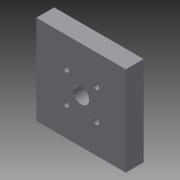
# Autodesk Inventor part: lmk8uugen
Saved by Autodesk Inventor 2014 (Build 180170000, 170)
## iProperties
Created: 2014-07-13
Part Number: lmk8uugen
Material: Generic
Document SubType Name: Modeling
Designer: cruiser
Density: 1 g/cm^3
Appearance: Default
Author: cruiser
Autodesk Inventor part; units mm, degrees
ref_plane "YZ Plane" through (0, 0, 0) normal (1, 0, 0) x (0, 1, 0)
ref_plane "XZ Plane" through (0, 0, 0) normal (0, 1, 0) x (-1, 0, 0)
ref_plane "XY Plane" through (0, 0, 0) normal (0, 0, 1) x (1, 0, 0)
sketch "Sketch1" plane through (0, 0, 0) normal (0, 1, 0) x (-1, 0, 0)
  line L0 (25, -25) -> (-25, -25)
  line L1 (-25, -25) -> (-25, 25)
  line L2 (-25, 25) -> (25, 25)
  line L3 (25, 25) -> (25, -25)
  line L4 (25, -25) -> (-25, 25) construction
  line L5 (-25, -25) -> (25, 25) construction
  point P0 (0, 0)
  dimension "d0" = 50
  dimension "d1" = 50
  constraints: 12 end point, 2 midpoint, 2 parallel, 1 horizontal, 1 perpendicular
  measures "d0" distance of L1.end L2.end
  measures "d1" distance of L0.end L1.end
extrude "Extrusion1" add sketch "Sketch1" along normal blind 10
sketch "Sketch2" plane through (0, 10, 0) normal (0, 1, 0) x (1, 0, 0)
  circle A0 centre (0, 0) radius 4.5
  circle A1 centre (8.4853, 8.4853) radius 1.65
  line L0 (0, 0) -> (8.4853, 8.4853)
  line L1 (0, 0) -> (12, 0) construction
  circle A2 centre (-8.4853, 8.4853) radius 1.65
  circle A3 centre (-8.4853, -8.4853) radius 1.65
  circle A4 centre (8.4853, -8.4853) radius 1.65
  dimension "d4" = 9
  dimension "d5" = 3.3
  dimension "d7" = 12
  dimension "d8" = 45
  dimension "d11" = 360
  constraints: 5 centre point, 4 end point, 2 coincident, 1 equal length, 1 horizontal, 9 other
  measures "d4" diameter of A0
  measures "d5" diameter of A1
  measures "d7" distance of L0.start L0.end
  measures "d8" angle of L1 L0
extrude "lmk8uu holes" cut sketch "Sketch2" against normal up to next
equation "\"d4\" = center_hole"
equation "\"d5\" = mount_hole"
equation "\"d7\" = hole_radius"
equation "\"hole_radius\" = 12"
equation "\"mount_hole\" = 3.3"
equation "\"center_hole\" = 9"
body "Solid1"
